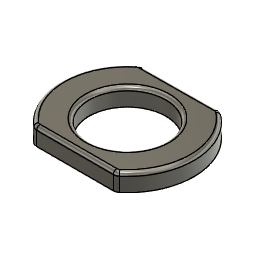
SpacerBlankingPlate v1 (Autodesk Fusion 360 design; units mm, degrees)
Autodesk Fusion 360 part; units mm, degrees
note: some values were not read from the file. Set by a fixed rule: which sketch regions a step uses.
sketch "Sketch1" plane through (0, 0, 0) normal (0, 1, 0) x (1, 0, 0)
  line L0 (0, 0) -> (-15, 0)
  line L1 (0, 0) -> (15, 0)
  circle A0 centre (15, 0) radius 3
  circle A1 centre (-15, 0) radius 3
  circle A2 centre (15, 0) radius 4
  circle A3 centre (-15, 0) radius 4
  circle A4 centre (0, 0) radius 11
  circle A5 centre (0, 0) radius 19
  line L2 (0, 0) -> (0, -15)
  line L3 (0, 0) -> (0, 15)
  line L4 (0, -15) -> (20.2663, -15)
  line L5 (20.2663, -15) -> (-18, -15)
  line L6 (0, 15) -> (-22, 15)
  line L7 (-22, 15) -> (21.8454, 15.4076)
  dimension "d1" = 15
  dimension "d2" = 15
  dimension "d3" = 6
  dimension "d4" = 6
  dimension "d5" = 8
  dimension "d6" = 8
  dimension "d7" = 38
  dimension "d8" = 15
  dimension "d9" = 15
  constraint coincident L0.start L1.start
  constraint horizontal L0
  constraint parallel L0 L1
  constraint coincident L1.end A0.centre
  constraint coincident L0.end A1.centre
  constraint concentric A0 A2
  constraint concentric A1 A3
  constraint tangent A2 A4
  constraint tangent A2 A5
  constraint perpendicular L0 L2
  constraint perpendicular L0 L3
  constraint perpendicular L2 L4
  constraint perpendicular L2 L5
  constraint perpendicular L3 L6
  measures "d1" distance of L0.start L0.end
  measures "d2" distance of L0.start L1.end
  measures "d3" diameter of A0
  measures "d4" diameter of A1
  measures "d5" diameter of A2
  measures "d6" diameter of A3
  measures "d7" diameter of A5
  measures "d8" distance of L0.start L2.end
  measures "d9" distance of L0.start L3.end
extrude "Extrude1" add sketch "Sketch1" along normal blind 5 contours A3 | A3 A4 A5 L2 L5 | A3 A4 A5 L3 L6 | A2 A4 A5 L3 L6 L7 | A2 | A2 A4 A5 L2 L4 L5 | A0 | A1
extrude "Extrude2" cut sketch "Sketch1" along normal blind 3.7 contours A0 | A1
fillet "Fillet1" radius 2 2 faces at (16.9556, 3.7, 0.2948) (-15.2176, 3.7, -0.9086)
fillet "Fillet2" radius 1 2 edges at (12.203, 0, 1.0848) (-17.797, 0, 1.0848)
fillet "Fillet3" radius 2 4 edges at (-11.6619, 2.5, 15) (11.6619, 2.5, 15) (-11.5357, 2.5, -15.0973) (11.253, 2.5, -15.3091)
fillet "Fillet4" radius 1 1 faces at (-0.3682, 5, -13.7919)
